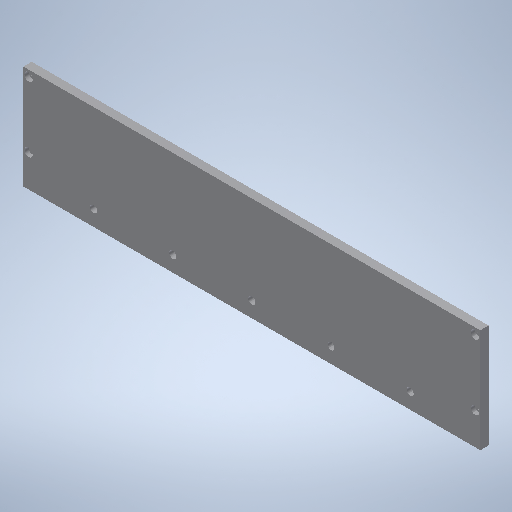
# Autodesk Inventor part: Bottom
Saved by Autodesk Inventor 2025 (Build 290162000, 162)
## iProperties
Created: 2010-12-14
Part Number: Bottom
Document SubType Name: Modeling
Designer: berny
Density: 2.7 g/cm^3
Material: Aluminum-6061
Mass: 787.603 g
Surface Area: 1009.94 cm^2
Volume: 291.705 cm^3
Appearance: Aluminum - Flat
Author: berny
Autodesk Inventor part; units mm, degrees
ref_plane "YZ Plane" through (0, 0, 0) normal (1, 0, 0) x (0, 1, 0)
ref_plane "XZ Plane" through (0, 0, 0) normal (0, 1, 0) x (-1, 0, 0)
ref_plane "XY Plane" through (0, 0, 0) normal (0, 0, 1) x (1, 0, 0)
sketch "Sketch1" plane through (0, 0, 0) normal (0, 0, 1) x (1, 0, 0)
  line L0 (0, 0) -> (440, 0)
  line L1 (440, 0) -> (440, 100)
  line L2 (440, 100) -> (0, 100)
  line L3 (0, 100) -> (0, 0)
  dimension "d0" = 100
  dimension "d1" = 440
  constraints: 8 end point, 2 parallel, 1 horizontal, 1 perpendicular
  measures "d0" distance of L2.end L0.start
  measures "d1" distance of L0.start L0.end
extrude "Extrusion1" add sketch "Sketch1" along normal blind 8
sketch "Sketch2" plane through (0, 0, 8) normal (0, 0, 1) x (1, 0, 0)
  line L0 (0, 0) -> (0, 100) projected
  line L1 (440, 100) -> (440, 0) projected
  line L2 (0, 100) -> (440, 100) projected
  point P0 (435, 31)
  point P1 (435, 94)
  point P2 (5, 31)
  point P3 (5, 94)
  dimension "d5" = 6
  dimension "d6" = 5
  dimension "d7" = 5
  dimension "d46" = 69
  constraints: 2 horizontal alignment, 2 vertical alignment
  measures "d5" vertical distance of L1.start point (435, 94)
  measures "d6" distance from line of L1 point (435, 31)
  measures "d7" distance from line of L0 point (5, 31)
  measures "d46" distance from line of point (435, 31) L2
hole "Hole1" at (435, 31, 8) at (435, 94, 8) at (5, 31, 8) at (5, 94, 8) direction (0, 0, -1) diameter 4.3 end through all counterbore diameter 8 counterbore depth 4 clearance for "Socket Head Cap Screw" size "M4" standard "Ansi Metric M Profile"
sketch "Sketch3" plane through (0, 0, 0) normal (0, 0, -1) x (-1, 0, 0)
  line L0 (0, 0) -> (-440, 0) projected
  line L1 (0, 100) -> (0, 0) projected
  point P0 (-67.6, 15)
  point P1 (-143.8, 15)
  point P2 (-220, 15)
  point P3 (-296.2, 15)
  point P4 (-372.4, 15)
  dimension "d15" = 67.6
  dimension "d16" = 15
  dimension "d40" = 76.2
  dimension "d45" = 440
  constraints: 1 horizontal, 4 other
  measures "d15" distance from line of point (-67.6, 15) L1
  measures "d16" distance from line of L0 point (-67.6, 15)
  measures "d40" distance of point (-67.6, 15) point (-143.8, 15)
  measures "d45" distance of L0.start L0.end
hole "Hole2" at (67.6, 15, 0) at (143.8, 15, 0) at (220, 15, 0) at (296.2, 15, 0) at (372.4, 15, 0) direction (0, 0, 1) diameter 6.7564 end through all counterbore diameter 11.1252 counterbore depth 3.81 clearance for "Socket Head Cap Screw" size "1/4" standard "Ansi Unified Screw Threads"
equation "\"d7\" = d6"
body "Solid1"
